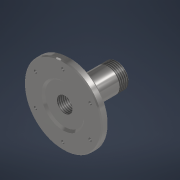
# Autodesk Inventor part: TUERCA DE TORNILLO DE ELEVACIÓN
Saved by Autodesk Inventor 2022 (Build 260153000, 153)
## iProperties
Created: 2021-09-20
Part Number: TUERCA DE TORNILLO DE ELEVACIÓN
Material: Steel, Alloy
Document SubType Name: Modeling
Designer: Andres
Density: 7.73 g/cm^3
Appearance: Semi-Polished
Author: Andres
Autodesk Inventor part; units mm, degrees
ref_plane "YZ Plane" through (0, 0, 0) normal (1, 0, 0) x (0, 1, 0)
ref_plane "XZ Plane" through (0, 0, 0) normal (0, 1, 0) x (-1, 0, 0)
ref_plane "XY Plane" through (0, 0, 0) normal (0, 0, 1) x (1, 0, 0)
sketch "Sketch1" plane through (0, 0, 0) normal (1, 0, 0) x (0, 1, 0)
  line L0 (0, -68.5665) -> (0, 42.4294) projected
  line L1 (0, 26.5728) -> (0, -52.7099)
  line L2 (-18, 2) -> (-18, -8)
  line L3 (-18, -8) -> (-12.5, -8)
  line L4 (-12.5, -8) -> (-12.5, -46)
  line L5 (-12.5, -46) -> (0, -46)
  line L6 (-18, 2) -> (-40, 2)
  line L7 (-40, 2) -> (-40, 10)
  line L8 (-40, 10) -> (0, 10)
  line L9 (-65, 0) -> (58.66, 0) projected
  line L10 (-65, 10) -> (58.66, 10) projected
  line L11 (-8, 10) -> (-8, -12)
  line L12 (-8, -12) -> (-9, -12)
  line L13 (-9, -12) -> (-9, -46)
  line L14 (-20, 8) -> (-8, 8)
  line L15 (-8, 8) -> (-8, 10)
  line L16 (-20, 8) -> (-20, 10)
  point P0 (0, 0)
  dimension "d1" = 80
  dimension "d2" = 2
  dimension "d3" = 8
  dimension "d4" = 25
  dimension "d5" = 36
  dimension "d11" = 16
  dimension "d16" = 8
  dimension "d17" = 38
  dimension "d50" = 1
  dimension "d57" = 34
  dimension "d63" = 2
  dimension "d64" = 40
  constraints: 28 end point, 8 perpendicular, 7 point on line, 3 vertical, 1 horizontal
  measures "d1" diameter of L7 L1
  measures "d2" distance between parallel lines of L6 L9
  measures "d3" distance between parallel lines of L6 L8
  measures "d4" diameter of L4 L1
  measures "d5" diameter of L2 L1
  measures "d11" diameter of L11 L1
  measures "d16" distance between parallel lines of L9 L3
  measures "d17" distance between parallel lines of L3 L5
  measures "d50" distance between parallel lines of L11 L13
  measures "d57" distance between parallel lines of L5 L12
  measures "d63" distance between parallel lines of L8 L14
  measures "d64" diameter of L16 L1
revolve "Revolution1" add sketch "Sketch1" angle 360 about axis through (0, 0, 26.5728) along (0, 0, -1) contours L5 L4 L3 L2 L9 L11 L12 L13 | L9 L2 L6 L7 L8 L16 L14 L11
chamfer "Chamfer1" distance 8 angle 30 1 edges at (0, 18, 2) measured on face at (0, 18, 1.5)
chamfer "Chamfer2" distance 2 angle 45 1 edges at (0, 40, 2)
sketch "Sketch2" plane through (0, 0, 10) normal (0, 0, 1) x (1, 0, 0)
  circle A0 centre (0, 0) radius 32.5 construction
  point P0 (0, -32.5)
  point P1 (28.1458, -16.25)
  point P2 (28.1458, 16.25)
  point P3 (0, 32.5)
  point P4 (-28.1458, 16.25)
  point P5 (-28.1458, -16.25)
  dimension "d24" = 65
  dimension "d27" = 360
  constraints: 2 vertical alignment, 1 coincident, 9 other
hole "Hole1" at (0, -32.5, 10) at (28.1458, -16.25, 10) at (28.1458, 16.25, 10) at (0, 32.5, 10) at (-28.1458, 16.25, 10) at (-28.1458, -16.25, 10) direction (0, 0, -1) diameter 3.242 depth 11.8 tip angle 118 thread size "M4x0.7" class "6H" standard "ISO Metric profile"
chamfer "Chamfer3" distance 1 angle 45 1 edges at (0, 9, -12)
chamfer "Chamfer5" distance 1 angle 45 1 edges at (0, 40, 10)
thread "Thread2" size "M16x2" class "6H" standard "ANSI Metric M Profile" full length
chamfer "Chamfer6" distance 2 angle 45 1 edges at (0, 20, 10)
thread "Thread3" size "M25x2" class "6g" standard "ISO Metric profile" length 10
chamfer "Chamfer7" distance 1 angle 45 1 edges at (0, 12.5, -46)
fillet "Fillet1" radius 0.5 1 edges at (0, 12.5, -8)
body "Solid1"
